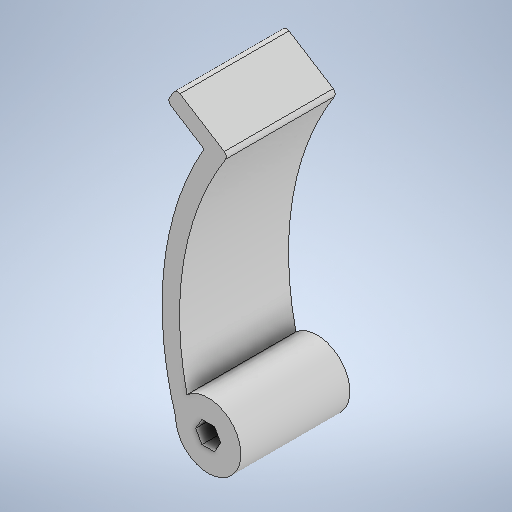
# Autodesk Inventor part: Pincer
Saved by Autodesk Inventor 2025.1 (Build 291241000, 241)
## iProperties
Created: 2024-12-07
Part Number: Pincer
Material: Generic
Document SubType Name: Modeling
Designer: ishaa
Density: 1 g/cm^3
Appearance: Default
Author: ishaa
Autodesk Inventor part; units mm, degrees
ref_plane "YZ Plane" through (0, 0, 0) normal (1, 0, 0) x (0, 1, 0)
ref_plane "XZ Plane" through (0, 0, 0) normal (0, 1, 0) x (-1, 0, 0)
ref_plane "XY Plane" through (0, 0, 0) normal (0, 0, 1) x (1, 0, 0)
sketch "Sketch1" plane through (0, 0, 0) normal (0, 0, 1) x (1, 0, 0)
  circle A0 centre (0, 0) radius 7.5
  arc A1 (-0.9428, 56.4732) -> (-7.5, -0.0097) centre (60.7261, 20.6919) ccw
  line L0 (-0.9428, 56.4732) -> (-8.5948, 61.2942)
  arc A2 (3.9984, 56.8989) -> (-3.6723, 1.1517) centre (60.7261, 20.6919) ccw
  line L1 (3.6885, 58.283) -> (-6.4626, 64.6785)
  line L2 (-8.9079, 62.6733) -> (-7.8417, 64.3655)
  arc A3 (-6.4626, 64.6785) -> (-7.8417, 64.3655) centre (-6.9957, 63.8324) ccw
  arc A4 (-8.9079, 62.6733) -> (-8.5948, 61.2942) centre (-8.0618, 62.1402) ccw
  arc A5 (3.9984, 56.8989) -> (3.6885, 58.283) centre (3.1555, 57.4369) ccw
  point P0 (-7.5, -0.0097)
  point P1 (4.546, 57.7428)
  point P2 (-4.8795, 5.6957)
  dimension "d0" = 15
  dimension "d11" = 4
  dimension "d12" = 1
  constraints: 13 point on circle, 6 centre point, 6 end point, 6 tangent, 2 equal radius, 1 coincident, 1 point on line, 1 other
  measures "d0" diameter of A0
  measures "d11" radial gap between concentric circles of A1 A2
  measures "d12" radius of A3
extrude "Extrusion1" add sketch "Sketch1" along normal blind 25
sketch "Sketch2" plane through (0, 0, 25) normal (0, 0, 1) x (1, 0, 0)
  line L0 (1.4434, 2.5) -> (2.8868, 0)
  line L1 (2.8868, 0) -> (1.4434, -2.5)
  line L2 (1.4434, -2.5) -> (-1.4434, -2.5)
  line L3 (-1.4434, -2.5) -> (-2.8868, 0)
  line L4 (-2.8868, 0) -> (-1.4434, 2.5)
  line L5 (-1.4434, 2.5) -> (1.4434, 2.5)
  point P0 (0, 0)
  point P1 (0, 0)
  dimension "d7" = 5
  constraints: 12 end point, 1 coincident, 13 other
  measures "d7" distance between parallel lines of L2 L5
extrude "Extrusion2" cut sketch "Sketch2" against normal blind 25
body "Solid1"
